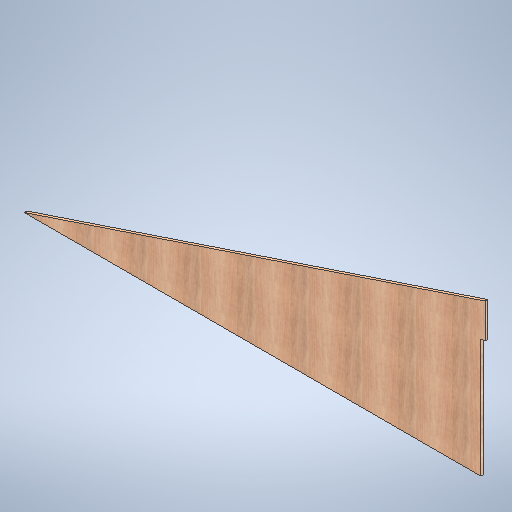
# Autodesk Inventor part: OSB_For_Side_And_Top
Saved by Autodesk Inventor 2025 (Build 290162010, 162A)
## iProperties
Created: 2024-09-19
Part Number: OSB_For_Side_And_Top
Material: Wood (Birch)
Document SubType Name: Modeling
Designer: Tom
Density: 0.55 g/cm^3
Appearance: Birch - Natural Polished
Author: Tom
Autodesk Inventor part; units mm, degrees
ref_plane "YZ Plane" through (0, 0, 0) normal (1, 0, 0) x (0, 1, 0)
ref_plane "XZ Plane" through (0, 0, 0) normal (0, 1, 0) x (-1, 0, 0)
ref_plane "XY Plane" through (0, 0, 0) normal (0, 0, 1) x (1, 0, 0)
sketch "Sketch1" plane through (0, 0, 0) normal (0, 0, 1) x (1, 0, 0)
  line L0 (0, 0) -> (0, 761.0602)
  line L1 (0, 0) -> (1219.2, 0)
  line L2 (0, 761.0602) -> (3365.5, 1883.9848)
  line L3 (12.7, 765.2977) -> (12.7, 0)
  line L4 (3365.5, 1883.9848) -> (3365.5, 1736.7138)
  line L5 (3365.5, 1736.7138) -> (101.6, 647.6888)
  line L6 (101.6, 647.6888) -> (12.7, 647.6888)
  line L7 (1219.2, 0) -> (1219.2, 1167.8555)
  line L8 (0, 761.0602) -> (-33.4963, 749.8839)
  line L9 (-33.4963, 749.8839) -> (-33.4963, 647.6888)
  line L10 (-33.4963, 647.6888) -> (0, 647.6888)
  line L11 (-33.4963, 749.8839) -> (-38.5208, 764.9428)
  line L12 (-38.5208, 764.9428) -> (1219.2, 1184.5909)
  line L13 (1219.2, 1184.5909) -> (1219.2, 1167.8555)
  line L14 (1219.2, 1184.5909) -> (3378.2, 1184.5909)
  line L15 (3378.2, 1184.5909) -> (3378.2, 0)
  line L16 (3378.2, 0) -> (1219.2, 0)
  line L17 (3365.5, 1883.9848) -> (3397.4278, 1894.6378)
  line L18 (3397.4278, 1894.6378) -> (3397.4278, 1747.3667)
  line L19 (3365.5, 1736.7138) -> (3397.4278, 1747.3667)
  line L20 (3397.4278, 1747.3667) -> (3365.5, 1747.3667)
  line L21 (1219.2, 1184.5909) -> (3397.4278, 1911.3731)
  line L22 (3397.4278, 1911.3731) -> (3397.4278, 1894.6378)
  line L23 (3378.2, 1184.5909) -> (3378.2, 1747.3667)
  line L24 (3378.2, 1747.3667) -> (3397.4278, 1747.3667)
  line L25 (3397.4278, 1747.3667) -> (3397.4278, 1894.6378)
  dimension "d1" = 761.0602
  dimension "d3" = 12.7
  dimension "d4" = 3352.8
  dimension "d6" = 139.7
  dimension "d8" = 88.9
  dimension "d9" = 1089.025
  dimension "d12" = 46.1962
  dimension "d14" = 15.875
  dimension "d16" = 1219.2
  dimension "d17" = 2159
  dimension "d20" = 31.9278
  constraints: 52 end point, 8 collinear, 8 vertical, 7 point on line, 5 horizontal, 3 parallel, 2 perpendicular
  measures "d1" distance of L0.start L0.end
  measures "d3" distance between parallel lines of L3 L0
  measures "d4" distance from line of L3 L2.end
  measures "d6" distance between parallel lines of L2 L5
  measures "d8" horizontal distance of L3.start L5.end
  measures "d9" vertical distance of L4.end L5.end
  measures "d12" distance between parallel lines of L9 L3
  measures "d14" distance between parallel lines of L2 L12
  measures "d16" distance of L0.start L1.end
  measures "d17" distance of L15.end L1.end
  measures "d20" distance between parallel lines of L18 L4
extrude "Extrusion1" add sketch "Sketch1" along normal blind 12.7 contours L14 L2 L4 L5 | L5 L19 L23 L14 | L14 L21 L22 L17 L2 | L4 L20 L23 L19 | L17 L18 L20 L4
body "Solid1"
